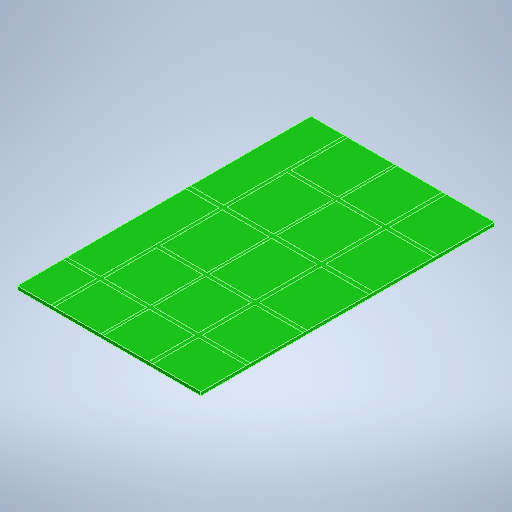
# Autodesk Inventor part: Placa
Saved by Autodesk Inventor 2025.2 (Build 292293000, 293)
## iProperties
Created: 2025-03-01
Part Number: Placa
Material: Genérico
Document SubType Name: Modeling
Designer: hmont
Density: 1 g/cm^3
Appearance: Verde oscuro
Author: hmont
Autodesk Inventor part; units mm, degrees
ref_plane "YZ Plane" through (0, 0, 0) normal (1, 0, 0) x (0, 1, 0)
ref_plane "XZ Plane" through (0, 0, 0) normal (0, 1, 0) x (-1, 0, 0)
ref_plane "XY Plane" through (0, 0, 0) normal (0, 0, 1) x (1, 0, 0)
sketch "Boceto1" plane through (0, 0, 0) normal (0, 1, 0) x (-1, 0, 0)
  line L0 (0, 0) -> (500, 0)
  line L1 (500, 0) -> (500, -800)
  line L2 (500, -800) -> (0, -800)
  line L3 (0, -800) -> (0, 0)
  dimension "d0" = 500
  dimension "d1" = 800
  constraints: 8 end point, 2 parallel, 1 horizontal, 1 perpendicular
  measures "d0" distance of L1.end L2.end
  measures "d1" distance of L0.end L1.end
extrude "Extrusión1" add sketch "Boceto1" along normal blind 10
sketch "Boceto3" plane through (0, 10, 0) normal (0, 1, 0) x (1, 0, 0)
  line L0 (0, 800) -> (-500, 800) projected
  line L1 (-500, 0) -> (0, 0) projected
  line L2 (-408.7792, 800) -> (-399.7054, 800)
  line L3 (-399.7054, 800) -> (-399.7054, 0)
  line L4 (-399.7054, 0) -> (-408.7792, 0)
  line L5 (-408.7792, 0) -> (-408.7792, 800)
  line L6 (-272.6715, 800) -> (-265.4124, 800)
  line L7 (-265.4124, 800) -> (-265.4124, 0)
  line L8 (-265.4124, 0) -> (-272.6715, 0)
  line L9 (-272.6715, 0) -> (-272.6715, 800)
  line L10 (-142.008, 800) -> (-131.1193, 800)
  line L11 (-131.1193, 800) -> (-131.1193, 0)
  line L12 (-131.1193, 0) -> (-142.008, 0)
  line L13 (-142.008, 0) -> (-142.008, 800)
  line L14 (-500, 800) -> (-500, 0) projected
  line L15 (0, 0) -> (0, 800) projected
  line L16 (-500, 645.1947) -> (0, 645.1947)
  line L17 (0, 645.1947) -> (0, 634.3061)
  line L18 (0, 634.3061) -> (-500, 634.3061)
  line L19 (-500, 634.3061) -> (-500, 645.1947)
  line L20 (-500, 470.9767) -> (0, 470.9767)
  line L21 (0, 470.9767) -> (0, 458.2733)
  line L22 (0, 458.2733) -> (-500, 458.2733)
  line L23 (-500, 458.2733) -> (-500, 470.9767)
  line L24 (-500, 289.4996) -> (0, 289.4996)
  line L25 (0, 289.4996) -> (0, 278.611)
  line L26 (0, 278.611) -> (-500, 278.611)
  line L27 (-500, 278.611) -> (-500, 289.4996)
  line L28 (-500, 135.2441) -> (0, 135.2441)
  line L29 (0, 135.2441) -> (0, 124.3555)
  line L30 (0, 124.3555) -> (-500, 124.3555)
  line L31 (-500, 124.3555) -> (-500, 135.2441)
  point P0 (-399.7054, 645.1947)
  point P1 (-408.7792, 634.3061)
  point P2 (-408.7792, 470.9767)
  point P3 (-408.7792, 458.2733)
  point P4 (-408.7792, 135.2441)
  point P5 (-408.7792, 124.3555)
  point P6 (-399.7054, 124.3555)
  point P7 (-272.6715, 124.3555)
  point P8 (-265.4124, 124.3555)
  point P9 (-142.008, 124.3555)
  point P10 (-131.1193, 124.3555)
  point P11 (0, 135.2441)
  point P12 (-131.1193, 135.2441)
  point P13 (-131.1193, 278.611)
  point P14 (0, 289.4996)
  point P15 (-131.1193, 289.4996)
  point P16 (-131.1193, 458.2733)
  point P17 (0, 470.9767)
  point P18 (-131.1193, 470.9767)
  point P19 (-131.1193, 634.3061)
  point P20 (0, 645.1947)
  point P21 (-131.1193, 645.1947)
  point P22 (-142.008, 645.1947)
  point P23 (-265.4124, 645.1947)
  point P24 (-272.6715, 645.1947)
  point P25 (-265.4124, 634.3061)
  point P26 (-142.008, 634.3061)
  point P27 (-142.008, 470.9767)
  point P28 (-265.4124, 470.9767)
  point P29 (-272.6715, 458.2733)
  point P30 (-272.6715, 289.4996)
  point P31 (-399.7054, 289.4996)
  point P32 (-399.7054, 458.2733)
  point P33 (-272.6715, 278.611)
  point P34 (-272.6715, 135.2441)
  point P35 (-399.7054, 135.2441)
  point P36 (-399.7054, 278.611)
  point P37 (-142.008, 278.611)
  point P38 (-142.008, 135.2441)
  point P39 (-265.4124, 135.2441)
  point P40 (-265.4124, 278.611)
  point P41 (-142.008, 458.2733)
  point P42 (-142.008, 289.4996)
  point P43 (-265.4124, 289.4996)
  point P44 (-265.4124, 458.2733)
  point P45 (-399.7054, 634.3061)
  point P46 (-272.6715, 634.3061)
  point P47 (-272.6715, 470.9767)
  point P48 (-399.7054, 470.9767)
  constraints: 56 end point, 14 parallel, 14 point on line, 7 horizontal, 7 perpendicular
extrude "Extrusión3" add sketch "Boceto3" along normal blind 0.1 contours L11 L16 L13 L0 | L15 L18 L11 L16 | L11 L18 L13 L16 | L7 L16 L9 L0 | L13 L18 L7 L16 | L11 L20 L13 L18 | L15 L22 L11 L20 | L7 L18 L9 L16 | L11 L22 L13 L20 | L3 L16 L5 L0 | L9 L18 L3 L16 | L7 L20 L9 L18 | L13 L22 L7 L20 | L11 L24 L13 L22 | L15 L26 L11 L24 | L3 L18 L5 L16 | L7 L22 L9 L20 | L11 L26 L13 L24 | L3 L20 L5 L18 | L9 L22 L3 L20 | L7 L24 L9 L22 | L13 L26 L7 L24 | L11 L28 L13 L26 | L15 L30 L11 L28 | L3 L22 L5 L20 | L7 L26 L9 L24 | L11 L30 L13 L28 | L5 L22 L14 L20 | L3 L24 L5 L22 | L9 L26 L3 L24 | L7 L28 L9 L26 | L13 L30 L7 L28 | L11 L1 L13 L30 | L3 L26 L5 L24 | L7 L30 L9 L28 | L3 L28 L5 L26 | L9 L30 L3 L28 | L7 L1 L9 L30 | L3 L30 L5 L28 | L5 L30 L14 L28 | L3 L1 L5 L30
